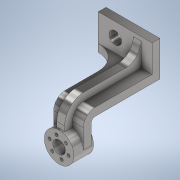
# Autodesk Inventor part: Кронштейн
Saved by Autodesk Inventor 2021 (Build 250183000, 183)
## iProperties
Created: 2020-10-15
Part Number: Кронштейн
Material: Сталь, высокопрочная, низколегированная
Document SubType Name: Modeling
Designer: User
Density: 7.85 g/cm^3
Appearance: Сталь — полированная
Author: User
Autodesk Inventor part; units mm, degrees
ref_plane "YZ Plane" through (0, 0, 0) normal (1, 0, 0) x (0, 1, 0)
ref_plane "XZ Plane" through (0, 0, 0) normal (0, 1, 0) x (-1, 0, 0)
ref_plane "XY Plane" through (0, 0, 0) normal (0, 0, 1) x (1, 0, 0)
sketch "Эскиз1" plane through (0, 0, 0) normal (0, 0, 1) x (1, 0, 0)
  line L0 (19, 0) -> (-50, 0)
  line L1 (-50, 0) -> (-50, 45)
  line L2 (-50, 45) -> (19, 45)
  line L3 (19, 45) -> (19, 0)
  point P0 (0, 0)
  dimension "d0" = 69
  dimension "d1" = 45
  dimension "d2" = 19
  constraints: 8 end point, 2 parallel, 1 horizontal, 1 horizontal alignment, 1 perpendicular
  measures "d0" distance of L1.end L2.end
  measures "d1" distance of L0.end L1.end
  measures "d2" distance of point (0, 0) L0.start
extrude "Выдавливание1" add sketch "Эскиз1" along normal blind 10
sketch "Эскиз2" plane through (19, 0, 0) normal (1, 0, 0) x (0, 0, -1)
  line L0 (-10, 45) -> (-10, 0) projected
  line L1 (-10, 10) -> (-98, 10)
  line L2 (-98, 10) -> (-98, -30)
  line L3 (-98, -30) -> (-88, -30)
  line L4 (-88, -30) -> (-88, 0)
  line L5 (0, 0) -> (-10, 0) projected
  line L6 (-88, 0) -> (-10, 0)
  dimension "d5" = 10
  dimension "d6" = 10
  dimension "d7" = 78
  dimension "d8" = 75
  constraints: 10 end point, 4 perpendicular, 1 collinear, 1 point on line
  measures "d5" distance between parallel lines of L2 L4
  measures "d6" distance between parallel lines of L6 L1
  measures "d7" horizontal distance of L3.end L0.end
  measures "d8" vertical distance of L2.end L0.start
extrude "Выдавливание2" add sketch "Эскиз2" against normal blind 38
fillet "Сопряжение1" radius 15 1 edges at (0, 10, 98)
fillet "Сопряжение1" radius 5 1 edges at (0, 0, 88)
fillet "Сопряжение1" radius 31 1 edges at (-19, 5, 10)
sketch "Эскиз3" plane through (-19, -30, 98) normal (0, 0, 1) x (1, 0, 0)
  line L0 (38, 0) -> (0, 0) construction
  circle A0 centre (19, 0) radius 19
  point P0 (19, 30)
  constraints: 1 horizontal alignment, 1 midpoint, 2 other
extrude "Выдавливание3" add sketch "Эскиз3" along normal blind 12 and the other way blind 13
sketch "Эскиз7" plane through (0, 0, 0) normal (1, 0, 0) x (0, 1, 0)
  line L0 (10, 10) -> (45, 10) construction
  line L1 (20, 10) -> (20, 108)
  line L2 (20, 108) -> (-11, 108)
  line L3 (-11, 85) -> (-11, 110) construction
  line L4 (10, 10) -> (10, 83) construction
  line L5 (-5, 98) -> (-30, 98) construction
  point P0 (0, 0)
  dimension "d46" = 10
  dimension "d47" = 10
  constraints: 4 end point, 2 perpendicular, 2 point on line
  measures "d46" distance between parallel lines of L4 L1
  measures "d47" distance between parallel lines of L2 L5
extrude "Ребро жесткости1" add sketch "Эскиз7" along normal mid plane 10 rib yes fills toward (19.95, 59) open curves L1 L2
fillet "Сопряжение2" radius 25 1 edges at (0, 20, 108)
fillet "Сопряжение2" radius 20 1 edges at (0, 20, 10)
sketch "Эскиз4" plane through (0, -30, 110) normal (0, 0, 1) x (1, 0, 0)
  arc A0 (19, 0) -> (-19, 0) centre (0, 0) ccw projected
  line L0 (0, 0) -> (8.8388, 8.8388)
  line L1 (0, 0) -> (12.5, 0) construction
  point P0 (0, 30)
  dimension "d18" = 12.5
  dimension "d19" = 45
  constraints: 4 end point, 1 equal length, 1 horizontal
  measures "d18" distance of L0.start L0.end
  measures "d19" angle of L1 L0
hole "Отверстие1" at (8.8388, -21.1612, 110) direction (0, 0, -1) diameter 4 end through all
pattern_circular "Круговой массив1" count 6 over 360 about axis through (0, -30, 98) along (0, 0, 1) of "Отверстие1"
sketch "Эскиз5" plane through (0, -30, 110) normal (0, 0, 1) x (1, 0, 0)
  circle A0 centre (0, 0) radius 19 projected
  point P0 (0, 30)
  constraints: 1 coincident
hole "Отверстие2" at (0, -30, 110) direction (0, 0, -1) diameter 16 end through all
sketch "Эскиз6" plane through (0, 0, 10) normal (0, 0, 1) x (1, 0, 0)
  line L0 (19, 45) -> (-50, 45) projected
  line L1 (-50, 45) -> (-50, 10) projected
  point P0 (0, 0)
  point P1 (-28, 27)
  dimension "d37" = 18
  dimension "d38" = 22
  measures "d37" distance from line of L0 point (-28, 27)
  measures "d38" distance from line of L1 point (-28, 27)
hole "Отверстие3" at (-28, 27, 10) direction (0, 0, -1) diameter 16 end through all
